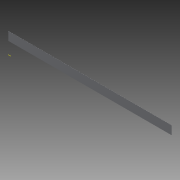
# Autodesk Inventor part: Cloth
Saved by Autodesk Inventor 2013 (Build 170138000, 138)
## iProperties
Created: 2014-01-18
Part Number: Cloth
Material: Generic
Document SubType Name: Modeling
Designer: 215152
Density: 1 g/cm^3
Author: 215152
Autodesk Inventor part; units mm, degrees
ref_plane "YZ Plane" through (0, 0, 0) normal (1, 0, 0) x (0, 1, 0)
ref_plane "XZ Plane" through (0, 0, 0) normal (0, 1, 0) x (-1, 0, 0)
ref_plane "XY Plane" through (0, 0, 0) normal (0, 0, 1) x (1, 0, 0)
ref_plane "Work Plane1" through (0, 37.5357, 0) normal (0, 0, 1) x (1, 0, 0)
sketch "Sketch1" plane through (0, 37.5357, 0) normal (0, 0, 1) x (1, 0, 0)
  line L0 (0, -37.5357) -> (482.346, -37.5357)
  line L1 (482.346, -37.5357) -> (482.346, -62.9357)
  line L2 (482.346, -62.9357) -> (0, -62.9357)
  line L3 (0, -62.9357) -> (0, -37.5357)
  line L4 (0, -62.9357) -> (0, -56.5857)
  line L5 (0, -56.5857) -> (482.346, -56.5857)
  line L6 (482.346, -56.5857) -> (482.346, -81.9857)
  line L7 (482.346, -81.9857) -> (0, -81.9857)
  line L8 (0, -81.9857) -> (0, -56.5857)
  dimension "d0" = 482.346
  dimension "d1" = 25.4
  dimension "d2" = 6.35
  dimension "d3" = 482.346
  dimension "d4" = 25.4
  constraints: 18 end point, 4 parallel, 2 horizontal, 2 perpendicular, 1 point on line
  measures "d0" distance of L1.end L2.end
  measures "d1" distance of L0.end L1.end
  measures "d2" distance of L2.end L4.end
  measures "d3" distance of L6.end L7.end
  measures "d4" distance of L5.end L6.end
extrude "Extrusion1" add sketch "Sketch1" along normal blind 0.254 contours L5 L1 L2 L3 | L2 L6 L7 L8
sketch "Sketch2" plane through (0, -44.45, 0) normal (-1, 0, 0) x (0, 0, 1)
  line L0 (0, 25.4) -> (0, 0) projected
  line L1 (0, 0) -> (0.254, 0) projected
  line L2 (0.254, 25.4) -> (0.254, 0) projected
  line L3 (0, 25.4) -> (0.254, 25.4) projected
  point P0 (0, 44.45)
extrude "Extrusion2" add sketch "Sketch2" along normal blind 0.254
sketch "Sketch3" plane through (482.346, -44.45, 0) normal (1, 0, 0) x (0, 0, -1)
  line L0 (0, 0) -> (0, 25.4) projected
  line L1 (0, 25.4) -> (-0.254, 25.4) projected
  line L2 (-0.254, 0) -> (-0.254, 25.4) projected
  line L3 (0, 0) -> (-0.254, 0) projected
  point P0 (0, 44.45)
extrude "Extrusion3" add sketch "Sketch3" along normal blind 0.254
sketch "Sketch4" plane through (0, 37.5357, 0) normal (0, 0, -1) x (-1, 0, 0)
  line L0 (-482.6, -56.5857) -> (-482.346, -56.5857)
  line L1 (-482.346, -56.5857) -> (-482.346, -81.9857)
  line L2 (-482.346, -81.9857) -> (-482.6, -81.9857)
  line L3 (-482.6, -81.9857) -> (-482.6, -56.5857)
  line L4 (0.254, -56.5857) -> (0, -56.5857)
  line L5 (0, -56.5857) -> (0, -81.9857)
  line L6 (0, -81.9857) -> (0.254, -81.9857)
  line L7 (0.254, -81.9857) -> (0.254, -56.5857)
  point P0 (0, -37.5357)
  dimension "d11" = 0.254
  dimension "d12" = 25.4
  dimension "d13" = 0.254
  dimension "d14" = 25.4
  constraints: 16 end point, 4 parallel, 2 horizontal, 2 perpendicular
  measures "d11" distance of L1.end L2.end
  measures "d12" distance of L0.end L1.end
  measures "d13" distance of L6.end L5.end
  measures "d14" distance of L5.end L4.end
extrude "Extrusion4" add sketch "Sketch4" along normal blind 25.4
body "Solid1"
